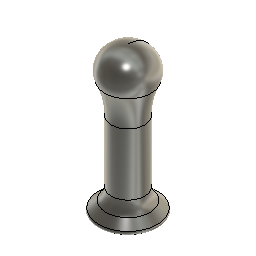
Joystick_ver2_rev_1.2 (Autodesk Fusion 360 design; units mm, degrees)
Autodesk Fusion 360 part; units mm, degrees
note: some values were not read from the file. Set by a fixed rule: which sketch regions a step uses.
sketch "Schizzo1" plane through (0, 0, 0) normal (1, 0, 0) x (0, 1, 0)
  line L0 (3.225, 0) -> (3.225, 15)
  line L1 (15.8979, -3.483) -> (21.2628, -8.3935)
  line L2 (20.25, -9.5) -> (21.75, -9.5) construction
  arc A0 (12.1624, 5) -> (15.8979, -3.483) centre (23.6624, 5) ccw
  line L3 (0, 0) -> (3.225, 0) construction
  line L4 (0, 0) -> (0, 15) construction
  line L5 (3.225, 15) -> (0, 15)
  line L6 (0, 95) -> (0, 15)
  line L7 (20.25, -11) -> (20.25, -9.5) construction
  line L8 (0, 95) -> (-15, 95) construction
  line L9 (12.1624, 5) -> (12.1624, 50)
  ellipse E0 centre (0, 78.5258) end of major axis (18.2065, 78.5258) minor radius 16.4742 (16.9001, 72.398) -> (0, 95) ccw
  arc A1 (16.9001, 72.398) -> (12.1624, 50) centre (67.476, 50) ccw
  line L10 (0, 81) -> (18, 81) construction
  line L11 (3.225, 0) -> (17.033, -10.788)
  arc A2 (20.25, -11) -> (21.2628, -8.3935) centre (20.25, -9.5) ccw
  line L12 (20.25, -11) -> (17.6487, -11)
  arc A3 (17.033, -10.788) -> (17.6487, -11) centre (17.6487, -10) ccw
  point P0 (11, 1)
  dimension "d1" = 3.225
  dimension "d2" = 15
  dimension "d6" = 3
  dimension "d7" = 21.75
  dimension "d8" = 11
  dimension "d9" = 1
  dimension "d24" = 11.5
  dimension "d38" = 90
  dimension "d41" = 4
  dimension "d45" = 18
  dimension "d46" = 14
  dimension "d47" = 45
  dimension "d48" = 1
  dimension "d49" = 142
  dimension "d50" = 11
  constraint vertical L0
  constraint perpendicular L0 L5
  constraint coincident L3.start L4.start
  constraint perpendicular L4 L5
  constraint perpendicular L0 L3
  constraint coincident L7.start A2.start
  constraint coincident L2.start L7.end
  constraint vertical L7
  constraint coincident L2.end A2
  constraint perpendicular L2 L7
  constraint tangent L1 A2
  constraint perpendicular L5 L6
  constraint coincident P0 L1
  constraint tangent L1 A0
  constraint perpendicular L6 L8
  constraint tangent A0 L9
  constraint vertical L9
  constraint tangent E0 A1
  constraint coincident L6 E0.centre
  constraint tangent L8 E0
  constraint tangent L9 A1
  constraint coincident L6 L10.start
  constraint coincident E0 L10.end
  constraint horizontal L10
  constraint tangent L11 A3
  constraint tangent L12 A3
  measures "d1" distance of L0 L4
  measures "d2" distance of L0.end L0.start
  measures "d6" diameter of A2
  measures "d7" distance of L2.end L4
  measures "d8" distance of P0 L4
  measures "d9" vertical distance of P0 L0.start
  measures "d24" radius of A0
  measures "d38" distance of L8 A0.start
  measures "d41" vertical distance of P0 A0.start
  measures "d45" distance of L10.start L10.end
  measures "d46" distance of L8 L10
  measures "d47" distance of L8 L9.end
  measures "d48" radius of A3
  measures "d49" angle of L11 L12
  measures "d50" distance of L3 L12
revolve "Rivoluzione1" add sketch "Schizzo1" angle 360 about axis through (0, 0, 95) along (0, 0, -1)
chamfer "Smusso1" distance 0.5 angle 45 1 edges at (-3.0068, 1.1662, 0)
equation "d1 = larghezza_incastro_joystick / 2"
equation "d7 = ( 43.5 / 2 ) * 1 mm"
equation "d8 = ( 22 / 2 ) * 1 mm"
equation "altezza_joystick = 90 mm" comment "Modificare questovalore per aumentare o diminuire l'altezza del joystick. (Valore di default 90.00 mm)"
equation "larghezza_incastro_joystick = 6.45 mm" comment "Modificare questo valore per allargare o diminuire il foro dell'incastro del Joystick. (Valore di default 6.45 mm)"
equation "d38 = altezza_joystick"
named bodies: "joystick_2"
